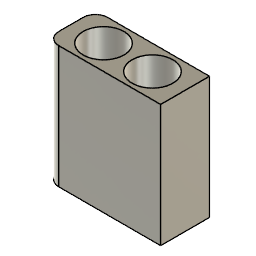
LED_holder_vert_v2 (Autodesk Fusion 360 design; units mm, degrees)
Autodesk Fusion 360 part; units mm, degrees
sketch "Skizze1" plane through (0, 0, 0) normal (0, 0, 1) x (1, 0, 0)
  circle A0 centre (-6, 0) radius 2.5
  circle A1 centre (0, 0) radius 2.5
  line L0 (0, 0) -> (4, 0)
  line L1 (4, 0) -> (4, 3)
  line L2 (4, 3) -> (-10, 3)
  line L3 (-10, 3) -> (-10, -3)
  line L4 (-10, -3) -> (4, -3)
  line L5 (4, -3) -> (4, 0)
  dimension "d1" = 5
  dimension "d2" = 5
  dimension "d3" = 6
  constraint coincident A1.centre L0.start
  constraint horizontal L0
  constraint perpendicular L0 L1
  constraint perpendicular L1 L2
  constraint perpendicular L2 L3
  constraint perpendicular L3 L4
  constraint perpendicular L0 L5
  measures "d1" diameter of A0
  measures "d2" diameter of A1
  measures "d3" distance of A1.centre A0.centre
extrude "Extrusion1" add sketch "Skizze1" along normal blind 10
fillet "Abrundung1" radius 1.5 2 edges at (-10, -3, 5) (-10, 3, 5)
extrude "Extrusion2" cut 1 faces at (3.5, 0, 10) along direction (0, 0, -1) blind 1
extrude "Extrusion3" add 1 faces at (3.5, 0, 9) along direction (0, 0, 1) blind 4
extrude "Extrusion4" add 1 faces at (3.5, 0, 13) along direction (0, 0, 1) blind 2
